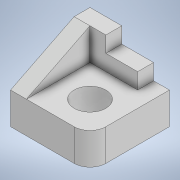
# Autodesk Inventor part: 件26
Saved by Autodesk Inventor 2020 (Build 240168000, 168)
## iProperties
Created: 2020-10-30
Part Number: 件26
Material: 一般
Document SubType Name: Modeling
Designer: USER
Density: 1 g/cm^3
Appearance: 預設
Author: USER
Autodesk Inventor part; units mm, degrees
ref_plane "YZ Plane" through (0, 0, 0) normal (1, 0, 0) x (0, 1, 0)
ref_plane "XZ Plane" through (0, 0, 0) normal (0, 1, 0) x (-1, 0, 0)
ref_plane "XY Plane" through (0, 0, 0) normal (0, 0, 1) x (1, 0, 0)
sketch "草圖1" plane through (0, 0, 0) normal (0, 0, 1) x (1, 0, 0)
  line L0 (25, -10) -> (-25, -10)
  line L1 (-25, -10) -> (-25, 10)
  line L2 (-25, 10) -> (25, 10)
  line L3 (25, 10) -> (25, -10)
  line L4 (25, -10) -> (-25, 10) construction
  line L5 (-25, -10) -> (25, 10) construction
  point P0 (0, 0)
  dimension "d0" = 20
  dimension "d1" = 50
  constraints: 12 end point, 2 midpoint, 2 parallel, 1 horizontal, 1 perpendicular
  measures "d0" distance between parallel lines of L0 L2
  measures "d1" distance between parallel lines of L3 L1
extrude "擠出1" add sketch "草圖1" along normal blind 50
sketch "草圖2" plane through (-25, 10, 0) normal (0, 1, 0) x (1, 0, 0)
  line L0 (0, 0) -> (40, 0)
  line L1 (40, 0) -> (40, -10)
  line L2 (40, -10) -> (0, -10)
  line L3 (0, -10) -> (0, 0)
  point P0 (25, 0)
  point P1 (0, 0)
  dimension "d6" = 40
  dimension "d7" = 10
  constraints: 8 end point, 2 parallel, 1 coincident, 1 horizontal, 1 perpendicular
  measures "d6" distance between parallel lines of L1 L3
  measures "d7" distance between parallel lines of L0 L2
extrude "擠出2" add sketch "草圖2" along normal blind 20
sketch "草圖3" plane through (-25, 10, 10) normal (0, 0, 1) x (1, 0, 0)
  line L0 (40, 20) -> (0, 20) projected
  line L1 (40, 20) -> (20, 20)
  line L2 (20, 20) -> (20, 10)
  line L3 (20, 10) -> (40, 10)
  line L4 (40, 10) -> (40, 20)
  line L5 (0, 0) -> (0, 20) projected
  line L6 (50, 0) -> (0, 0) projected
  point P0 (25, -10)
  dimension "d10" = 20
  dimension "d11" = 10
  constraints: 8 end point, 2 parallel, 1 horizontal, 1 perpendicular
  measures "d10" distance between parallel lines of L2 L5
  measures "d11" distance between parallel lines of L6 L3
extrude "擠出3" cut sketch "草圖3" against normal blind 20
sketch "草圖4" plane through (-25, -10, 50) normal (-1, 0, 0) x (0, 0, 1)
  line L0 (-40, 40) -> (-50, 40) projected
  line L1 (-50, 20) -> (0, 20) projected
  line L2 (-40, 40) -> (0, 20)
  line L3 (0, 20) -> (-40, 20)
  line L4 (-40, 20) -> (-40, 40)
  point P0 (-50, 10)
  constraints: 6 end point, 1 horizontal, 1 perpendicular
extrude "擠出4" add sketch "草圖4" against normal blind 10
sketch "草圖5" plane through (25, 10, 50) normal (0, 1, 0) x (1, 0, 0)
  circle A0 centre (-20, 20) radius 10
  line L0 (0, 0) -> (-40, 0) projected
  line L1 (0, 50) -> (0, 0) projected
  point P0 (-25, 50)
  dimension "d16" = 20
  dimension "d17" = 20
  dimension "d18" = 20
  constraints: 1 centre point
  measures "d16" distance from line of L0 A0.centre
  measures "d17" distance from line of L1 A0.centre
  measures "d18" diameter of A0
extrude "擠出5" cut sketch "草圖5" against normal blind 27.75
fillet "圓角1" radius 10 1 edges at (25, 0, 50)
